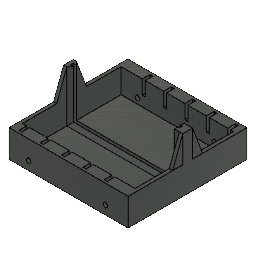
T_breakout_holder (Autodesk Fusion 360 design; units mm, degrees)
Autodesk Fusion 360 part; units mm, degrees
note: some values were not read from the file. Chosen so that the rebuilt part matches the saved one: which bodies a step acts on.
sketch "Sketch1" plane through (0, 0, 0) normal (0, 1, 0) x (1, 0, 0)
  line L0 (32.5, 7.25) -> (-32.5, 7.25)
  line L1 (-32.5, 7.25) -> (-32.5, -7.25)
  line L2 (-32.5, -7.25) -> (32.5, -7.25)
  line L3 (32.5, -7.25) -> (32.5, 7.25)
  line L4 (32.5, 7.25) -> (-32.5, -7.25) construction
  line L5 (-32.5, 7.25) -> (32.5, -7.25) construction
  circle A0 centre (22.76, -4.15) radius 1.27
  circle A1 centre (-22.975, -4.15) radius 1.27
  line L6 (18.06, 24.85) -> (19.81, 24.85)
  line L7 (19.81, 24.85) -> (19.81, -1.15)
  line L8 (19.81, -1.15) -> (18.06, -1.15)
  line L9 (18.06, -1.15) -> (18.06, 24.85)
  line L10 (5.36, -1.15) -> (5.36, 24.85)
  line L11 (5.36, 24.85) -> (7.11, 24.85)
  line L12 (7.11, -1.15) -> (5.36, -1.15)
  line L13 (7.11, 24.85) -> (7.11, -1.15)
  line L14 (-7.34, -1.15) -> (-7.34, 24.85)
  line L15 (-7.34, 24.85) -> (-5.59, 24.85)
  line L16 (-5.59, 24.85) -> (-5.59, -1.15)
  line L17 (-5.59, -1.15) -> (-7.34, -1.15)
  line L18 (-20.04, -1.15) -> (-20.04, 24.85)
  line L19 (-20.04, 24.85) -> (-18.29, 24.85)
  line L20 (-18.29, -1.15) -> (-20.04, -1.15)
  line L21 (-18.29, 24.85) -> (-18.29, -1.15)
  line L22 (-32.74, -1.15) -> (-32.74, 24.85)
  line L23 (-32.74, 24.85) -> (-30.99, 24.85)
  line L24 (-30.99, 24.85) -> (-30.99, -1.15)
  line L25 (-30.99, -1.15) -> (-32.74, -1.15)
  line L26 (-36.5, 7.25) -> (34.5, 7.25)
  line L27 (34.5, 7.25) -> (34.5, -9.25)
  line L28 (34.5, -9.25) -> (-36.5, -9.25)
  line L29 (-36.5, -9.25) -> (-36.5, 7.25)
  line L30 (-36.5, 7.25) -> (-34.5, 7.25)
  line L31 (-34.5, 7.25) -> (-34.5, -9.25)
  line L32 (-34.5, -9.25) -> (-36.5, -9.25)
  line L33 (-36.5, -9.25) -> (-36.5, 7.25)
  line L34 (-32.5, -7.25) -> (-34.5, -7.25)
  dimension "d3" = 65
  dimension "d4" = 14.5
  dimension "d5" = 2.54
  dimension "d6" = 2.54
  dimension "d7" = 3.1
  dimension "d8" = 3.1
  dimension "d9" = 9.74
  dimension "d10" = 45.735
  dimension "d11" = 26
  dimension "d12" = 1.75
  dimension "d13" = 4.7
  dimension "d14" = 3
  dimension "d15" = 26
  dimension "d16" = 1.75
  dimension "d17" = 26
  dimension "d18" = 1.75
  dimension "d19" = 26
  dimension "d20" = 1.75
  dimension "d21" = 26
  dimension "d22" = 1.75
  dimension "d23" = 71
  dimension "d24" = 16.5
  dimension "d25" = 2
  dimension "d26" = 4
  dimension "d27" = 2
  constraint perpendicular L0 L1
  constraint parallel L0 L2
  constraint parallel L1 L3
  constraint horizontal L0
  constraint coincident L4 origin
  constraint coincident L5 origin
  constraint horizontal L6
  constraint vertical L7
  constraint horizontal L8
  constraint vertical L9
  constraint horizontal L11
  constraint vertical L13
  constraint horizontal L12
  constraint vertical L10
  constraint horizontal L15
  constraint vertical L16
  constraint horizontal L17
  constraint vertical L14
  constraint horizontal L19
  constraint vertical L21
  constraint horizontal L20
  constraint vertical L18
  constraint horizontal L23
  constraint vertical L24
  constraint horizontal L25
  constraint vertical L22
  constraint horizontal L26
  constraint vertical L27
  constraint horizontal L28
  constraint vertical L29
  constraint horizontal L30
  constraint vertical L31
  constraint horizontal L32
  constraint vertical L33
  constraint coincident L28 L31.end
  constraint coincident L31 L34.end
  constraint perpendicular L31 L34
  measures "d3" distance of L1.end L2.end
  measures "d4" distance of L0.end L1.end
  measures "d5" diameter of A0
  measures "d6" diameter of A1
  measures "d7" distance of L2 A0.centre
  measures "d8" distance of L2 A1.centre
  measures "d9" distance of L3 A0.centre
  measures "d10" distance of A0.centre A1.centre
  measures "d11" distance of L6.start L8.end
  measures "d12" distance of L6.start L6.end
  measures "d13" distance of A0.centre L9
  measures "d14" distance of A0.centre L8
  measures "d15" distance of L10.start L10.end
  measures "d16" distance of L11.end L10.end
  measures "d17" distance of L14.start L14.end
  measures "d18" distance of L15.end L14.end
  measures "d19" distance of L18.end L18.start
  measures "d20" distance of L18.end L19.end
  measures "d21" distance of L22.end L22.start
  measures "d22" distance of L23.end L22.end
  measures "d23" distance of L26.start L26.end
  measures "d24" distance of L26.start L28.end
  measures "d25" distance of L2 L28
  measures "d26" distance of L1 L29
  measures "d27" distance of L26.start L30.end
extrude "Extrude3" add sketch "Sketch1" along normal blind 1.5 contours L0 L1 L2 L3 L7 L8 L9 L10 L12 L13 L14 L16 L17 L18 L20 L21 L24 L25 L26 | L2 L3 L26 L27 L28 L31 L34 | L0 L7 L8 L9 L26 | L1 L22 L25 L26 L31 L34 | L0 L10 L12 L13 L26 | L1 L22 L25 L26 | L0 L1 L24 L25 L26 | L26 L28 L29 L30 L31 L32 L33 | L0 L14 L16 L17 L26 | L0 L18 L20 L21 L26 | A0 | A1 makes body 1
extrude "Extrude2" add sketch "Sketch1" against normal blind 33 separate body contours L2 L3 L26 L27 L28 L31 L34 | L26 L28 L29 L30 L31 L32 L33 makes body 2
extrude "Extrude1" add sketch "Sketch1" against normal blind 4.572 separate body contours L0 L1 L2 L3 L7 L8 L9 L10 L12 L13 L14 L16 L17 L18 L20 L21 L24 L25 L26 | L2 L3 L26 L27 L28 L31 L34 | L1 L22 L25 L26 L31 L34 | L26 L28 L29 L30 L31 L32 L33 makes body 3
sketch "Sketch2" plane through (-34.5, 0, 0) normal (1, 0, 0) x (0, 0, -1)
  line L0 (-7.25, 0) -> (-7.25, -33)
  line L1 (-7.25, -33) -> (7.25, -33)
  line L2 (7.25, -33) -> (7.25, 0)
  line L3 (-7.25, -33) -> (-5.25, -33)
  line L4 (-5.25, -33) -> (-7.25, -31)
  line L5 (-5.25, -33) -> (-2.4216, -33) construction
  line L6 (-7.25, -31) -> (-7.25, -33)
  line L7 (7.25, 0) -> (-7.25, 0)
  dimension "d34" = 135
  constraint coincident L0.end L1.start
  constraint perpendicular L0 L3
  constraint coincident L0 L4.end
  constraint horizontal L5
  measures "d34" angle of L4 L5
extrude "Extrude4" add sketch "Sketch2" along normal up to surface (67 mm away) separate body contours L0 L1 L3 L4 L6 makes body 4
sketch "Sketch4" plane through (0, 0, 7.25) normal (0, 0, -1) x (-1, 0, 0)
  line L0 (-32.5, 0) -> (-32.5, -33)
  line L1 (-32.5, -33) -> (34.5, -33)
  line L2 (34.5, -33) -> (34.5, 0)
  line L3 (32.5, 0) -> (32.5, -33)
  line L4 (-32.5, -33) -> (-30.5, -33)
  line L5 (-30.5, -33) -> (-32.5, -31)
  line L6 (-30.5, -33) -> (-27.6716, -33) construction
  line L7 (-32.5, -31) -> (-32.5, -33)
  line L8 (32.5, -33) -> (31, -33)
  line L9 (31, -33) -> (32.5, -31.5)
  line L10 (32.5, -31.5) -> (34.5, -31.5)
  line L11 (34.5, -31.5) -> (34.5, -33)
  line L12 (34.5, -33) -> (32.5, -33)
  line L13 (32.5, -33) -> (32.5, -31.5)
  line L14 (34.5, 0) -> (-32.5, 0)
  line L15 (32.5, -31) -> (34.5, -31)
  line L16 (34.5, -31) -> (34.5, -33)
  line L17 (34.5, -33) -> (32.5, -33)
  line L18 (32.5, -33) -> (32.5, -31)
  line L19 (32.5, -31) -> (31.5, -31)
  line L20 (31.5, -31) -> (31.5, -33)
  line L21 (31.5, -33) -> (32.5, -33)
  line L22 (32.5, -33) -> (32.5, -31)
  line L23 (31.5, -31) -> (34.5, -28)
  line L24 (31.5, -31) -> (35.7426, -31) construction
  line L25 (34.5, -31) -> (34.5, -28)
  dimension "d37" = 33
  dimension "d38" = 2
  dimension "d39" = 135
  dimension "d40" = 1.5
  dimension "d41" = 45
  dimension "d84" = 45
  constraint coincident L0.end L1.start
  constraint perpendicular L0 L4
  constraint coincident L0 L5.end
  constraint horizontal L6
  constraint perpendicular L3 L8
  constraint coincident L3 L9.end
  constraint horizontal L10
  constraint vertical L11
  constraint horizontal L12
  constraint vertical L13
  constraint coincident L1.end L2.start
  constraint horizontal L15
  constraint vertical L16
  constraint horizontal L17
  constraint vertical L18
  constraint coincident L3 L15.start
  constraint horizontal L19
  constraint vertical L20
  constraint horizontal L21
  constraint vertical L22
  constraint coincident L8 L20.end
  constraint coincident L1 L20.end
  constraint coincident L2 L23.end
  constraint horizontal L24
  measures "d37" distance of L3.start L3.end
  measures "d38" distance of L0.end L4.end
  measures "d39" angle of L5 L6
  measures "d40" distance of L3.end L8.end
  measures "d41" angle of L6 L9
  measures "d84" angle of L23 L24
extrude "Extrude5" add sketch "Sketch4" along normal blind 14.5 separate body contours L0 L1 L4 L5 L7 | L2 L3 L15 L23 L25 | L3 L19 L23 | L1 L8 L9 L20 | L2 L3 L10 L15 L16 L18 L22 | L3 L9 L18 L19 L20 L22 | L1 L3 L8 L9 L13 L18 L20 L21 L22 | L1 L2 L3 L10 L11 L12 L13 L16 L17 L18 L22 makes body 5 at (-34.5, -31.3333, -2.4167) makes body 6 at (31.1667, -32.3333, 2.4167)
sketch "Sketch5" plane through (0, -33, 0) normal (0, -1, 0) x (1, 0, 0)
  line L0 (-34.5, 7.25) -> (32.5, 7.25)
  line L1 (32.5, 7.25) -> (32.5, -7.25)
  line L2 (32.5, -7.25) -> (34.5, -7.25)
  line L3 (34.5, -7.25) -> (34.5, 9.25)
  line L4 (34.5, 9.25) -> (-36.5, 9.25)
  line L5 (-36.5, 9.25) -> (-36.5, -7.25)
  line L6 (-36.5, -7.25) -> (-34.5, -7.25)
  line L7 (-34.5, -7.25) -> (-34.5, 7.25)
  line L8 (-36.5, -7.25) -> (-32.5, -7.25)
  line L9 (-32.5, -7.25) -> (-32.5, 9.25)
  line L10 (-32.5, 9.25) -> (-36.5, 9.25)
  line L11 (-36.5, 9.25) -> (-36.5, -7.25)
  dimension "d46" = 4
  dimension "d47" = 16.5
  constraint horizontal L8
  constraint vertical L9
  constraint horizontal L10
  constraint vertical L11
  constraint coincident L5.end L6.start
  measures "d46" distance of L5.end L8.end
  measures "d47" distance of L5.end L4.end
extrude "Extrude6" add sketch "Sketch5" along normal blind 0.9 separate body makes body 7
sketch "Sketch9" plane through (0, 0, -7.25) normal (0, 0, -1) x (-1, 0, 0)
  line L0 (-32.5, 0) -> (-34.5, 0)
  line L1 (-34.5, 0) -> (-34.5, -33)
  line L2 (-34.5, -33) -> (-32.5, -33)
  line L3 (-32.5, -33) -> (-32.5, 0)
  line L4 (-34.5, -33.9) -> (36.5, -33.9)
  line L5 (-34.5, -33.9) -> (-32.5, -33.9)
  line L6 (-32.5, -33) -> (-30.5, -33)
  line L7 (-30.5, -33) -> (-32.5, -31)
  line L8 (-34.5, -31) -> (-34.5, -33.9)
  line L9 (-34.5, -31) -> (-32.5, -31)
  line L10 (-32.5, -33.9) -> (-32.5, -33)
  line L11 (31, -33) -> (32.5, -33)
  line L12 (32.5, -33) -> (32.5, -33.9)
  line L13 (32.5, -33.9) -> (36.5, -33.9)
  line L14 (31.5, -32.5) -> (31, -33)
  line L15 (31, -33) -> (32.2574, -31.7574)
  line L16 (32.5, -31) -> (32.5, -32)
  line L17 (36.5, 0) -> (36.5, -33)
  line L18 (32.5, -31) -> (36.5, -31)
  line L19 (36.5, -31) -> (36.5, -33.9)
  line L20 (32.2574, -31.7574) -> (32.5, -31.5)
  line L21 (32.6899, -32) -> (32.5, -32)
  line L22 (-32.5, -31) -> (34.5, -31)
  line L23 (31.5, -32.5) -> (31.5, -31)
  point P0 (-34.5, -33.9)
  point P1 (-32.5, -33.9)
  point P2 (-30.5, -33)
  point P3 (-32.5, -31)
  point P4 (31, -33)
  point P5 (32.5, -33)
  point P6 (32.5, -33.9)
  point P7 (32.5, -31)
  point P8 (31.5, -32.5)
  point P9 (31, -33)
  point P10 (31.5, -32.5)
  point P11 (31, -33)
  point P12 (31.5, -31)
  constraint coincident P0 L4.start
  constraint coincident P1 L5.end
  constraint coincident L2.end L3.start
  constraint coincident P2 L6.end
  constraint coincident P3 L7.end
  constraint coincident L1 L8.start
  constraint perpendicular L5 L8
  constraint perpendicular L3 L9
  constraint coincident P11 P9
  constraint coincident P5 L11.end
  constraint coincident P6 L12.end
  constraint coincident L4.end L13.end
  constraint coincident P7 L16.start
  constraint coincident L17 L18.end
  constraint perpendicular L16 L18
  constraint midpoint L16 L20.end
  constraint coincident P10 P8
  constraint coincident P12 L23.end
extrude "Extrude9" add sketch "Sketch9" along normal blind 16 separate body contours L3 L6 L7 | L1 L2 L3 L8 L9 | L2 L4 L5 L8 L10 | L14 L15 L16 L20 L22 L23 | L4 L11 L12 L13 L15 L16 L17 L18 L19 L20 L22 makes body 8 at (34.5, -31.9667, -12.5833) makes body 9 at (-33.8333, -31, -17.9167)
sketch "Sketch10" plane through (34.5, 0, 0) normal (1, 0, 0) x (0, 0, -1)
  line L0 (7.25, -31) -> (7.25, -33.9)
  line L1 (7.25, -33.9) -> (23.25, -33.9)
  line L2 (23.25, -33.9) -> (23.25, -31)
  line L3 (23.25, -31) -> (7.25, -31)
  line L4 (7.25, 0) -> (7.25, -33)
  line L5 (7.25, -31) -> (7.25, -25)
  line L6 (7.25, -25) -> (23.25, -31)
  line L7 (23.25, -31) -> (7.25, -31)
  constraint coincident L0.start L3.end
  constraint coincident L4 L5.end
  constraint perpendicular L3 L5
  constraint coincident L2.end L3.start
extrude "Extrude10" add sketch "Sketch10" against normal blind 2 separate body contours L3 L4 L5 L6 L7 makes body 10
sketch "Sketch11" plane through (-36.5, 0, 0) normal (-1, 0, 0) x (0, 0, 1)
  line L0 (-7.25, -33.9) -> (-7.25, -31)
  line L1 (-7.25, -31) -> (-23.25, -31)
  line L2 (-23.25, -31) -> (-23.25, -33.9)
  line L3 (-23.25, -33.9) -> (-7.25, -33.9)
  line L4 (-7.25, -31) -> (-7.25, -25)
  line L5 (-7.25, -25) -> (-23.25, -31)
  line L6 (-23.25, -31) -> (-7.25, -31)
  point P0 (-7.25, -25)
  constraint coincident L0.end L1.start
  constraint coincident P0 L4.end
  constraint coincident L1.end L2.start
extrude "Extrude11" add sketch "Sketch11" against normal blind 2 separate body contours L1 L4 L5 L6 makes body 11
mirror "Mirror1" about plane through (0, -33.9, 0) normal (0, -1, 0) of bodies 5 4 6 2 1 7 10 8 11 9 makes body 12 at (-12.1667, -35.4667, 5.9167) makes body 13 at (-32.5, -37.8, 2.4167) makes body 14 at (1.7867, -67.8, 3.75) makes body 15 at (-35.1667, -33.9, 3.0833) makes body 16 at (31.1667, -35.4667, 2.4167) makes body 17 at (11.5, -45.8, 9.25) makes body 18 at (34.5, -38.8, -12.5833) makes body 19 at (-36.5, -38.8, -12.5833) makes body 20 at (34.5, -35.8333, -12.5833) makes body 21 at (-33.8333, -36.8, -17.9167)
sketch "Sketch6" plane through (0, -4.572, 0) normal (0, -1, 0) x (1, 0, 0)
  circle A0 centre (22.76, 4.15) radius 1.27
  circle A1 centre (-22.975, 4.15) radius 1.27
  line L0 (19.81, 1.15) -> (19.81, -7.25)
  line L1 (19.81, -7.25) -> (34.5, -7.25)
  line L2 (34.5, -7.25) -> (34.5, 9.25)
  line L3 (34.5, 9.25) -> (-36.5, 9.25)
  line L4 (-36.5, 9.25) -> (-36.5, -7.25)
  line L5 (-36.5, -7.25) -> (-32.74, -7.25)
  line L6 (-32.74, -7.25) -> (-32.74, 1.15)
  line L7 (-32.74, 1.15) -> (-30.99, 1.15)
  line L8 (-30.99, 1.15) -> (-30.99, -7.25)
  line L9 (-30.99, -7.25) -> (-20.04, -7.25)
  line L10 (-20.04, -7.25) -> (-20.04, 1.15)
  line L11 (-20.04, 1.15) -> (-18.29, 1.15)
  line L12 (-18.29, 1.15) -> (-18.29, -7.25)
  line L13 (-18.29, -7.25) -> (-7.34, -7.25)
  line L14 (-7.34, -7.25) -> (-7.34, 1.15)
  line L15 (-7.34, 1.15) -> (-5.59, 1.15)
  line L16 (-5.59, 1.15) -> (-5.59, -7.25)
  line L17 (-5.59, -7.25) -> (5.36, -7.25)
  line L18 (5.36, -7.25) -> (5.36, 1.15)
  line L19 (5.36, 1.15) -> (7.11, 1.15)
  line L20 (7.11, 1.15) -> (7.11, -7.25)
  line L21 (7.11, -7.25) -> (18.06, -7.25)
  line L22 (18.06, -7.25) -> (18.06, 1.15)
  line L23 (18.06, 1.15) -> (19.81, 1.15)
  circle A2 centre (-22.975, 4.15) radius 1.27
  circle A3 centre (22.76, 4.15) radius 1.27
  dimension "d49" = 2.54
  dimension "d50" = 2.54
  constraint concentric A1 A2
  constraint concentric A0 A3
  measures "d49" diameter of A2
  measures "d50" diameter of A3
extrude "Extrude7" cut sketch "Sketch6" along normal blind 70 contours A0 A3 | A1 A2 bodies 4 14 12
sketch "Sketch7" plane through (0, -67.8, 0) normal (0, 1, 0) x (-1, 0, 0)
  circle A0 centre (-22.76, 4.15) radius 1.27
  circle A1 centre (22.975, 4.15) radius 1.27
  line L0 (36.5, 9.25) -> (-34.5, 9.25)
  line L1 (-34.5, 9.25) -> (-34.5, -7.25)
  line L2 (-34.5, -7.25) -> (36.5, -7.25)
  line L3 (36.5, -7.25) -> (36.5, 9.25)
  line L4 (-29.99, 1.15) -> (-28.24, 1.15)
  line L5 (-28.24, 1.15) -> (-28.24, -24.85)
  line L6 (-28.24, -24.85) -> (-29.99, -24.85)
  line L7 (-29.99, -24.85) -> (-29.99, 1.15)
  circle A2 centre (-22.76, 4.15) radius 1.27
  circle A3 centre (22.975, 4.15) radius 1.27
  line L8 (-15.54, 1.15) -> (-15.54, -24.85)
  line L9 (-15.54, -24.85) -> (-17.29, -24.85)
  line L10 (-17.29, -24.85) -> (-17.29, 1.15)
  line L11 (-17.29, 1.15) -> (-15.54, 1.15)
  line L12 (8.11, -24.85) -> (8.11, 1.15)
  line L13 (8.11, 1.15) -> (9.86, 1.15)
  line L14 (9.86, 1.15) -> (9.86, -24.85)
  line L15 (9.86, -24.85) -> (8.11, -24.85)
  line L16 (-4.59, -24.85) -> (-4.59, 1.15)
  line L17 (-4.59, 1.15) -> (-2.84, 1.15)
  line L18 (-2.84, -24.85) -> (-4.59, -24.85)
  line L19 (-2.84, 1.15) -> (-2.84, -24.85)
  line L20 (22.56, 1.15) -> (22.56, -24.85)
  line L21 (22.56, -24.85) -> (20.81, -24.85)
  line L22 (20.81, 1.15) -> (22.56, 1.15)
  line L23 (20.81, -24.85) -> (20.81, 1.15)
  line L24 (-34.5, 9.25) -> (36.5, 9.25)
  line L25 (36.5, 9.25) -> (36.5, -7.25)
  line L26 (36.5, -7.25) -> (-34.5, -7.25)
  line L27 (-34.5, -7.25) -> (-34.5, 9.25)
  dimension "d53" = 26
  dimension "d54" = 1.75
  dimension "d55" = 2.54
  dimension "d56" = 2.54
  dimension "d57" = 7.23
  dimension "d58" = 3
  dimension "d59" = 26
  dimension "d60" = 1.75
  dimension "d63" = 26
  dimension "d64" = 1.75
  dimension "d65" = 26
  dimension "d66" = 1.75
  dimension "d67" = 26
  dimension "d68" = 1.75
  constraint horizontal L4
  constraint vertical L5
  constraint horizontal L6
  constraint vertical L7
  constraint concentric A0 A2
  constraint concentric A1 A3
  constraint horizontal L11
  constraint vertical L8
  constraint horizontal L9
  constraint vertical L10
  constraint horizontal L17
  constraint vertical L19
  constraint horizontal L18
  constraint vertical L16
  constraint horizontal L13
  constraint vertical L14
  constraint horizontal L15
  constraint vertical L12
  constraint horizontal L22
  constraint vertical L20
  constraint horizontal L21
  constraint vertical L23
  constraint horizontal L24
  constraint vertical L25
  constraint horizontal L26
  constraint vertical L27
  constraint coincident L2.end L3.start
  constraint coincident L0.end L1.start
  measures "d53" distance of L4.start L6.end
  measures "d54" distance of L4.start L4.end
  measures "d55" diameter of A2
  measures "d56" diameter of A3
  measures "d57" distance of L7 A0.centre
  measures "d58" distance of L4 A0.centre
  measures "d59" distance of L9.end L10.end
  measures "d60" distance of L10.end L8.start
  measures "d63" distance of L16.start L16.end
  measures "d64" distance of L16.end L17.end
  measures "d65" distance of L12.start L12.end
  measures "d66" distance of L13.end L12.end
  measures "d67" distance of L22.start L21.end
  measures "d68" distance of L20.start L22.start
extrude "Extrude8" add sketch "Sketch7" along normal blind 4.572 separate body contours L0 L1 L2 L3 L4 L5 L7 L8 L10 L11 L12 L13 L14 L16 L17 L19 L20 L22 L23 L24 L25 L26 L27 makes body 22
sketch "Sketch8" plane through (0, 0, 0) normal (0, 1, 0) x (1, 0, 0)
combine "Combine1" operation add target body 22 tool bodies 14 10 21 9 19 20 11 18 8 2 12 6 5 13 4 7 15 1 16 3 17
sketch "Sketch12" plane through (0, -69.3, 0) normal (0, -1, 0) x (1, 0, 0)
  circle A0 centre (22.76, 4.15) radius 1.27
  circle A1 centre (-22.975, 4.15) radius 1.27
  line L0 (34.5, 9.25) -> (-36.5, 9.25)
  line L1 (-36.5, 9.25) -> (-36.5, -7.25)
  line L2 (-36.5, -7.25) -> (34.5, -7.25)
  line L3 (34.5, -7.25) -> (34.5, 9.25)
  line L4 (20.9641, 4.1753) -> (22.7347, 2.3541)
  line L5 (22.7347, 2.3541) -> (24.5559, 4.1247)
  line L6 (24.5559, 4.1247) -> (22.7853, 5.9459)
  line L7 (22.7853, 5.9459) -> (20.9641, 4.1753)
  line L8 (20.9641, 4.1753) -> (24.5559, 4.1247) construction
  line L9 (22.7347, 2.3541) -> (22.7853, 5.9459) construction
  circle A2 centre (22.76, 4.15) radius 1.27
  circle A3 centre (-22.975, 4.15) radius 1.27
  line L10 (-22.975, 2.3539) -> (-21.1789, 4.15)
  line L11 (-21.1789, 4.15) -> (-22.975, 5.9461)
  line L12 (-22.975, 5.9461) -> (-24.7711, 4.15)
  line L13 (-24.7711, 4.15) -> (-22.975, 2.3539)
  line L14 (-22.975, 2.3539) -> (-22.975, 5.9461) construction
  line L15 (-21.1789, 4.15) -> (-24.7711, 4.15) construction
  point P0 (22.76, 4.15)
  point P1 (-22.975, 4.15)
  dimension "d77" = 2.54
  dimension "d78" = 2.54
  dimension "d79" = 2.54
  dimension "d80" = 2.54
  constraint perpendicular L4 L5
  constraint parallel L4 L6
  constraint parallel L5 L7
  constraint coincident L8 P0
  constraint coincident L9 P0
  constraint coincident P0 A0.centre
  constraint concentric A1 A3
  constraint perpendicular L10 L11
  constraint parallel L10 L12
  constraint parallel L11 L13
  constraint coincident L14 P1
  constraint coincident L15 P1
  constraint coincident P1 A1.centre
  measures "d77" distance of L5.end L6.end
  measures "d78" distance of L4.end L5.end
  measures "d79" distance of L11.end L12.end
  measures "d80" distance of L10.end L11.end
extrude "Extrude12" cut sketch "Sketch12" against normal blind 200 contours A0 A2 | A0 L4 L5 A2 | A1 A3 | A1 A3 L10 L13 bodies 22
move_body "Move1" bodies 22 to x (1, 0, 0) y (0, 0, 1) z (0, -1, 0) at (0, -15.9594, 34.4594)
move_body "Move2" bodies 22 to x (-1, 0, 0) y (0, 1, 0) z (0, 0, -1) at (0, 0, 0)
